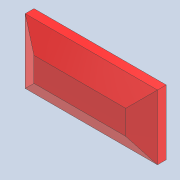
# Autodesk Inventor part: Pads
Saved by Autodesk Inventor 2022.3 (Build 263350030, 350C)
## iProperties
Created: 2022-11-01
Part Number: Pads
Material: Generic
Document SubType Name: Modeling
Designer: benka
Density: 1 g/cm^3
Appearance: Default
Author: benka
Autodesk Inventor part; units mm, degrees
ref_plane "YZ Plane" through (0, 0, 0) normal (1, 0, 0) x (0, 1, 0)
ref_plane "XZ Plane" through (0, 0, 0) normal (0, 1, 0) x (-1, 0, 0)
ref_plane "Work Plane1" through (-273.6, -145.5093, 1.1) normal (0, 0, 1) x (1, 0, 0)
sketch "Sketch1" plane through (0, 0, 0) normal (0, 0, 1) x (1, 0, 0)
  line L0 (-273.6, -142.1074) -> (-273.6, 15) projected
  line L1 (-273.6, -142.1074) -> (-273.5328, -142.3023) projected
  line L2 (-273.5328, -142.3023) -> (-271.5577, -145.5093) projected
  line L3 (-271.5577, -145.5093) -> (27.9577, -145.5093) projected
  line L4 (27.9577, -145.5093) -> (29.9328, -142.3023) projected
  line L5 (29.9328, -142.3023) -> (30, -142.1074) projected
  line L6 (30, -142.1074) -> (30, 15) projected
  line L7 (30, 15) -> (-273.6, 15) projected
  ellipse E0 centre (-207.1368, -126.3725) end of major axis (-207.1368, -124.9133) minor radius 1.45 (-205.7085, -126.6236) -> (-208.5652, -126.6236) ccw projected
  ellipse E1 centre (-207.1368, -126.8715) end of major axis (-205.6868, -126.8715) minor radius 1.4408 (-208.5652, -126.6236) -> (-205.7085, -126.6236) ccw projected
  line L8 (10, -5) -> (-10, -5) projected
  line L9 (-10, -5) -> (-10, 5) projected
  line L10 (-10, 5) -> (10, 5) projected
  line L11 (10, 5) -> (10, -5) projected
  line L12 (-131.8, -134.6879) -> (-131.8, -124.6879) projected
  line L13 (-131.8, -124.6879) -> (-111.8, -124.6879) projected
  line L14 (-111.8, -124.6879) -> (-111.8, -134.6879) projected
  line L15 (-111.8, -134.6879) -> (-131.8, -134.6879) projected
  line L16 (-233.6, -124.6879) -> (-233.6, -134.6879) projected
  line L17 (-233.6, -134.6879) -> (-253.6, -134.6879) projected
  line L18 (-253.6, -134.6879) -> (-253.6, -124.6879) projected
  line L19 (-253.6, -124.6879) -> (-233.6, -124.6879) projected
  line L20 (-131.8, -5) -> (-131.8, 5) projected
  line L21 (-131.8, 5) -> (-111.8, 5) projected
  line L22 (-111.8, 5) -> (-111.8, -5) projected
  line L23 (-111.8, -5) -> (-131.8, -5) projected
  line L24 (-10, -124.6879) -> (10, -124.6879) projected
  line L25 (10, -124.6879) -> (10, -134.6879) projected
  line L26 (10, -134.6879) -> (-10, -134.6879) projected
  line L27 (-10, -134.6879) -> (-10, -124.6879) projected
  line L28 (-233.6, 5) -> (-233.6, -5) projected
  line L29 (-233.6, -5) -> (-253.6, -5) projected
  line L30 (-253.6, -5) -> (-253.6, 5) projected
  line L31 (-253.6, 5) -> (-233.6, 5) projected
  ellipse E2 centre (-268.2527, 10.0167) end of major axis (-268.2527, 11.4759) minor radius 1.45 (-266.8028, 9.9997) -> (-269.7026, 9.9997) ccw projected
  ellipse E3 centre (-268.2527, 9.9828) end of major axis (-268.2527, 8.5236) minor radius 1.45 (-269.7026, 9.9997) -> (-266.8028, 9.9997) ccw projected
  ellipse E4 centre (25.0696, -126.3725) end of major axis (25.0696, -124.9133) minor radius 1.45 (26.5195, -126.3895) -> (23.6197, -126.3895) ccw projected
  ellipse E5 centre (25.0696, -126.4064) end of major axis (25.0696, -127.8656) minor radius 1.45 (23.6197, -126.3895) -> (26.5195, -126.3895) ccw projected
  ellipse E6 centre (-268.2527, -58.2135) end of major axis (-268.2527, -56.7542) minor radius 1.45 (-266.8028, -58.2304) -> (-269.7026, -58.2304) ccw projected
  ellipse E7 centre (-268.2527, -58.2474) end of major axis (-268.2527, -59.7066) minor radius 1.45 (-269.7026, -58.2304) -> (-266.8028, -58.2304) ccw projected
  ellipse E8 centre (-83.992, 10.0167) end of major axis (-83.992, 11.4759) minor radius 1.45 (-82.5421, 9.9997) -> (-85.4419, 9.9997) ccw projected
  ellipse E9 centre (-83.992, 9.9828) end of major axis (-83.992, 8.5236) minor radius 1.45 (-85.4419, 9.9997) -> (-82.5421, 9.9997) ccw projected
  ellipse E10 centre (25.0696, -58.2135) end of major axis (25.0696, -56.7542) minor radius 1.45 (26.5195, -58.2304) -> (23.6197, -58.2304) ccw projected
  ellipse E11 centre (25.0696, -58.2474) end of major axis (25.0696, -59.7066) minor radius 1.45 (23.6197, -58.2304) -> (26.5195, -58.2304) ccw projected
  ellipse E12 centre (-62.1557, -126.3725) end of major axis (-62.1557, -124.9133) minor radius 1.45 (-60.7058, -126.3895) -> (-63.6056, -126.3895) ccw projected
  ellipse E13 centre (-62.1557, -126.4064) end of major axis (-62.1557, -127.8656) minor radius 1.45 (-63.6056, -126.3895) -> (-60.7058, -126.3895) ccw projected
  ellipse E14 centre (-268.2527, -126.3725) end of major axis (-268.2527, -124.9133) minor radius 1.45 (-266.8028, -126.3895) -> (-269.7026, -126.3895) ccw projected
  ellipse E15 centre (-268.2527, -126.4064) end of major axis (-268.2527, -127.8656) minor radius 1.45 (-269.7026, -126.3895) -> (-266.8028, -126.3895) ccw projected
  ellipse E16 centre (-167.7791, 10.0167) end of major axis (-167.7791, 11.4759) minor radius 1.45 (-166.3292, 9.9997) -> (-169.229, 9.9997) ccw projected
  ellipse E17 centre (-167.7791, 9.9828) end of major axis (-167.7791, 8.5236) minor radius 1.45 (-169.229, 9.9997) -> (-166.3292, 9.9997) ccw projected
  ellipse E18 centre (-151.1416, -126.3725) end of major axis (-151.1416, -124.9133) minor radius 1.45 (-149.7132, -126.6236) -> (-152.5699, -126.6236) ccw projected
  ellipse E19 centre (-151.1416, -126.8715) end of major axis (-149.6916, -126.8715) minor radius 1.4408 (-152.5699, -126.6236) -> (-149.7132, -126.6236) ccw projected
  ellipse E20 centre (25.0696, 10.0167) end of major axis (25.0696, 11.4759) minor radius 1.45 (26.5195, 9.9997) -> (23.6197, 9.9997) ccw projected
  ellipse E21 centre (25.0696, 9.9828) end of major axis (25.0696, 8.5236) minor radius 1.45 (23.6197, 9.9997) -> (26.5195, 9.9997) ccw projected
  line L32 (-9.8, 4.8) -> (9.8, 4.8)
  line L33 (9.8, 4.8) -> (9.8, -4.8)
  line L34 (9.8, -4.8) -> (-9.8, -4.8)
  line L35 (-9.8, -4.8) -> (-9.8, 4.8)
  line L36 (-6.8, 1.8) -> (6.8, 1.8)
  line L37 (6.8, 1.8) -> (6.8, -1.8)
  line L38 (6.8, -1.8) -> (-6.8, -1.8)
  line L39 (-6.8, -1.8) -> (-6.8, 1.8)
  point P0 (0, 0)
  point P1 (0, 0)
  point P2 (-121.8, 0)
  point P3 (-243.6, 0)
  point P4 (-243.6, -129.6879)
  point P5 (-121.8, -129.6879)
  point P6 (0, -129.6879)
  point P7 (0, 0)
  dimension "d0" = 19.6
  dimension "d1" = 9.6
  dimension "d2" = 13.6
  dimension "d3" = 3.6
  constraints: 16 end point, 4 parallel, 2 horizontal, 2 perpendicular, 22 other
  measures "d0" distance of L33.end L34.end
  measures "d1" distance of L32.end L33.end
  measures "d2" distance of L37.end L38.end
  measures "d3" distance of L36.end L37.end
extrude "Extrusion1" add sketch "Sketch1" along normal blind 1.3 contours L32 L33 L34 L35 | L36 L37 L38 L39
sketch "Sketch2" plane through (0, 0, 1.3) normal (0, 0, 1) x (1, 0, 0)
  line L0 (-6.8, 1.8) -> (6.8, 1.8)
  line L1 (6.8, 1.8) -> (6.8, -1.8)
  line L2 (6.8, -1.8) -> (-6.8, -1.8)
  line L3 (-6.8, -1.8) -> (-6.8, 1.8)
  point P0 (0, 0)
  point P1 (0, 0)
  dimension "d6" = 13.6
  dimension "d7" = 3.6
  constraints: 8 end point, 2 parallel, 1 horizontal, 1 perpendicular
  measures "d6" distance of L1.end L2.end
  measures "d7" distance of L0.end L1.end
extrude "Extrusion2" add sketch "Sketch2" along normal blind 1.7
sketch "Sketch3" plane through (-9.8, -4.8, 0) normal (0, -1, 0) x (1, 0, 0)
  line L0 (16.6, 3) -> (3, 3) projected
  line L1 (0, 1.3) -> (3, 3)
  line L2 (3, 3) -> (16.6, 3)
  line L3 (19.6, 1.3) -> (0, 1.3) projected
  line L4 (16.6, 3) -> (19.6, 1.3)
  line L5 (0, 0) -> (0, 1.3) projected
  line L6 (19.6, 1.3) -> (0, 1.3)
  point P0 (9.8, 0)
  constraints: 8 end point, 1 collinear, 1 perpendicular
extrude "Extrusion3" add sketch "Sketch3" against normal up to surface (9.6 mm away)
sketch "Sketch4" plane through (9.8, -4.8, 0) normal (1, 0, 0) x (0, 0, -1)
  line L0 (0, 0) -> (-1.3, 0) projected
  line L1 (-1.3, 0) -> (-1.3, 3)
  line L2 (-1.3, 9.6) -> (-1.3, 0) projected
  line L3 (0, 9.6) -> (-1.3, 9.6) projected
  line L4 (-1.3, 9.6) -> (-1.3, 6.6)
  line L5 (-1.3, 0) -> (-3, 3)
  line L6 (-3, 0) -> (-3, 9.6) projected
  line L7 (-3, 6.6) -> (-1.3, 9.6)
  line L8 (-3, 0) -> (-1.3, 0) projected
  line L9 (-1.3, 0) -> (-3, 0)
  line L10 (-3, 0) -> (-3, 9.6)
  line L11 (-3, 9.6) -> (-1.3, 9.6) projected
  line L12 (-3, 9.6) -> (-1.3, 9.6)
  point P0 (0, 4.8)
  dimension "d12" = 3
  dimension "d13" = 3
  constraints: 14 end point, 3 point on line, 2 collinear, 1 perpendicular
  measures "d12" distance of L0.end L1.end
  measures "d13" distance of L2.start L4.end
extrude "Extrusion4" cut sketch "Sketch4" against normal through all contours L8 L6 L5 | L6 L11 L7
body "Solid1"
